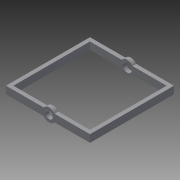
# Autodesk Inventor part: joystick_mount
Saved by Autodesk Inventor 2015 (Build 190159000, 159)
## iProperties
Created: 2015-12-08
Part Number: joystick_mount
Material: Generic
Document SubType Name: Modeling
Designer: boztalay
Density: 1 g/cm^3
Appearance: Default
Author: boztalay
Autodesk Inventor part; units mm, degrees
ref_plane "YZ Plane" through (0, 0, 0) normal (1, 0, 0) x (0, 1, 0)
ref_plane "XZ Plane" through (0, 0, 0) normal (0, 1, 0) x (-1, 0, 0)
ref_plane "XY Plane" through (0, 0, 0) normal (0, 0, 1) x (1, 0, 0)
sketch "Sketch1" plane through (0, 0, 0) normal (0, 1, 0) x (-1, 0, 0)
  line L0 (-63.5, 63.5) -> (63.5, 63.5)
  line L1 (63.5, 63.5) -> (63.5, -63.5)
  line L2 (63.5, -63.5) -> (-63.5, -63.5)
  line L3 (-63.5, -63.5) -> (-63.5, 63.5)
  line L4 (-63.5, 63.5) -> (63.5, -63.5) construction
  line L5 (63.5, 63.5) -> (-63.5, -63.5) construction
  line L6 (-69.85, 69.85) -> (69.85, 69.85)
  line L7 (69.85, 69.85) -> (69.85, -69.85)
  line L8 (69.85, -69.85) -> (-69.85, -69.85)
  line L9 (-69.85, -69.85) -> (-69.85, 69.85)
  line L10 (-69.85, 69.85) -> (69.85, -69.85) construction
  line L11 (69.85, 69.85) -> (-69.85, -69.85) construction
  point P0 (0, 0)
  dimension "d0" = 127
  dimension "d1" = 127
  dimension "d2" = 139.7
  dimension "d3" = 139.7
  constraints: 24 end point, 4 midpoint, 4 parallel, 2 horizontal, 2 perpendicular
  measures "d0" distance of L0.end L1.end
  measures "d1" distance of L1.end L2.end
  measures "d2" distance of L7.end L8.end
  measures "d3" distance of L6.end L7.end
extrude "Extrusion1" add sketch "Sketch1" along normal blind 12.7
sketch "Sketch2" plane through (69.85, 0, -69.85) normal (0, 0, -1) x (-1, 0, 0)
  circle A0 centre (69.85, 6.35) radius 11.1125
  line L0 (0, 0) -> (0, 12.7) construction
  line L1 (0, 6.35) -> (69.85, 6.35) construction
  line L2 (69.85, 6.35) -> (139.7, 6.35) construction
  line L3 (139.7, 0) -> (139.7, 12.7) construction
  point P0 (69.85, 0)
  dimension "d6" = 22.225
  constraints: 4 end point, 2 midpoint, 1 centre point, 1 collinear, 1 horizontal
  measures "d6" diameter of A0
extrude "Extrusion2" add sketch "Sketch2" against normal up to surface (6.35 mm away)
sketch "Sketch3" plane through (69.85, 0, -69.85) normal (0, 0, -1) x (-1, 0, 0)
  circle A0 centre (69.85, 6.35) radius 7.9375
  line L0 (0, 0) -> (0, 12.7) construction
  line L1 (0, 6.35) -> (69.85, 6.35) construction
  line L2 (69.85, 6.35) -> (139.7, 6.35) construction
  line L3 (139.7, 0) -> (139.7, 12.7) construction
  point P0 (69.85, 0)
  dimension "d9" = 15.875
  constraints: 4 end point, 2 midpoint, 1 centre point, 1 collinear, 1 horizontal
  measures "d9" diameter of A0
extrude "Extrusion3" cut sketch "Sketch3" against normal up to next
sketch "Sketch4" plane through (-69.85, 0, 69.85) normal (0, 0, 1) x (1, 0, 0)
  circle A0 centre (69.85, 6.35) radius 11.1125
  line L0 (0, 0) -> (0, 12.7) construction
  line L1 (0, 6.35) -> (69.85, 6.35) construction
  line L2 (69.85, 6.35) -> (139.7, 6.35) construction
  line L3 (139.7, 0) -> (139.7, 12.7) construction
  point P0 (69.85, 0)
  dimension "d12" = 22.225
  constraints: 4 end point, 2 midpoint, 1 centre point, 1 collinear, 1 horizontal
  measures "d12" diameter of A0
extrude "Extrusion4" add sketch "Sketch4" against normal up to surface (6.35 mm away)
sketch "Sketch5" plane through (-69.85, 0, 69.85) normal (0, 0, 1) x (1, 0, 0)
  circle A0 centre (69.85, 6.35) radius 6.35
  line L0 (0, 0) -> (0, 12.7) construction
  line L1 (0, 6.35) -> (69.85, 6.35) construction
  line L2 (69.85, 6.35) -> (139.7, 6.35) construction
  line L3 (139.7, 0) -> (139.7, 12.7) construction
  point P0 (69.85, 0)
  dimension "d15" = 12.7
  constraints: 4 end point, 2 midpoint, 1 centre point, 1 collinear, 1 horizontal
  measures "d15" diameter of A0
extrude "Extrusion5" cut sketch "Sketch5" against normal up to next
body "Solid1"
